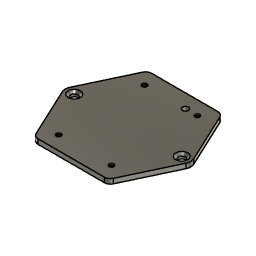
Metal Foot Pedal Bracket (Autodesk Fusion 360 design; units mm, degrees)
Autodesk Fusion 360 part; units mm, degrees
note: some values were not read from the file. Set by a fixed rule: which sketch regions a step uses.
sketch "Sketch1" plane through (0, 0, 0) normal (0, 0, 1) x (1, 0, 0)
  line L0 (22.1, 35.95) -> (-22.1, 35.95) construction
  line L1 (-22.1, 35.95) -> (-22.1, -35.95) construction
  line L2 (-22.1, -35.95) -> (22.1, -35.95) construction
  line L3 (22.1, -35.95) -> (22.1, 35.95) construction
  line L4 (22.1, 35.95) -> (-22.1, -35.95) construction
  line L5 (-22.1, 35.95) -> (22.1, -35.95) construction
  line L6 (23.8, 37.65) -> (-23.8, 37.65) construction
  line L7 (-23.8, 37.65) -> (-23.8, -37.65) construction
  line L8 (-23.8, -37.65) -> (23.8, -37.65) construction
  line L9 (23.8, -37.65) -> (23.8, 37.65) construction
  line L10 (23.8, 37.65) -> (-23.8, -37.65) construction
  line L11 (-23.8, 37.65) -> (23.8, -37.65) construction
  circle A0 centre (-22.1, 35.95) radius 1.7
  circle A1 centre (22.1, 35.95) radius 1.7
  circle A2 centre (-22.1, -35.95) radius 1.7
  circle A3 centre (22.1, -35.95) radius 1.7
  line L12 (-23.8, -34.25) -> (23.8, -34.25) construction
  line L13 (-20.4, -37.65) -> (-20.4, 37.65) construction
  line L14 (-23.8, 34.25) -> (23.8, 34.25) construction
  line L15 (20.4, 37.65) -> (20.4, -37.65) construction
  line L16 (31, 47.5) -> (-31, 47.5)
  line L17 (-31, 47.5) -> (-31, -47.5)
  line L18 (-31, -47.5) -> (31, -47.5)
  line L19 (31, -47.5) -> (31, 47.5)
  line L20 (31, 47.5) -> (-31, -47.5) construction
  line L21 (-31, 47.5) -> (31, -47.5) construction
  circle A4 centre (-45, 0) radius 3
  circle A5 centre (45, 0) radius 3
  circle A6 centre (-45, 0) radius 7.5
  circle A7 centre (45, 0) radius 7.5
  line L22 (-31, 47.5) -> (-51.7899, 3.1854)
  line L23 (-31, -47.5) -> (-51.7899, -3.1854)
  line L24 (31, -47.5) -> (51.7899, -3.1854)
  line L25 (31, 47.5) -> (51.7899, 3.1854)
  line L26 (45, 0) -> (0, 0) construction
  line L27 (0, 0) -> (-45, 0) construction
  circle A8 centre (12.1, 35.95) radius 2.5
  dimension "d1" = 75.3
  dimension "d2" = 68.5
  dimension "d3" = 40.8
  dimension "d4" = 47.6
  dimension "d5" = 95
  dimension "d6" = 62
  dimension "d7" = 6
  dimension "d8" = 6
  dimension "d9" = 15
  dimension "d10" = 15
  dimension "d11" = 45
  dimension "d12" = 45
  dimension "d13" = 10
  dimension "d14" = 5
  constraint horizontal L0
  constraint perpendicular L0 L1
  constraint parallel L0 L2
  constraint parallel L1 L3
  constraint coincident L4 L26.end
  constraint coincident L5 L26.end
  constraint coincident L26.end L27.start
  constraint horizontal L6
  constraint perpendicular L6 L7
  constraint parallel L6 L8
  constraint parallel L7 L9
  constraint coincident L10 L26.end
  constraint coincident L11 L26.end
  constraint coincident L0.end L1.start
  constraint coincident L0.start L3.end
  constraint coincident L1.end L2.start
  constraint coincident L2.end L3.start
  constraint tangent L8 A2
  constraint tangent L7 A2
  constraint tangent L8 A3
  constraint coincident L7 L12.start
  constraint coincident L9 L12.end
  constraint perpendicular L9 L12
  constraint coincident L8 L13.start
  constraint coincident L6 L13.end
  constraint coincident L7 L14.start
  constraint coincident L9 L14.end
  constraint perpendicular L9 L14
  constraint coincident L6 L15.start
  constraint coincident L8 L15.end
  constraint tangent A3 L15
  constraint vertical L15
  constraint tangent A1 L15
  constraint tangent L6 A1
  constraint tangent A1 L14
  constraint tangent A0 L14
  constraint tangent A0 L13
  constraint tangent A3 L12
  constraint tangent A2 L13
  constraint horizontal L16
  constraint perpendicular L16 L17
  constraint parallel L16 L18
  constraint parallel L17 L19
  constraint coincident L20 L26.end
  constraint coincident L21 L26.end
  constraint concentric A4 A6
  constraint concentric A5 A7
  constraint coincident A5.centre A7.centre
  constraint horizontal L26
  constraint coincident A4.centre A6.centre
  constraint parallel L26 L27
  constraint tangent A6 L22
  constraint tangent A6 L23
  constraint tangent A7 L24
  constraint tangent A7 L25
  constraint coincident A7 L25.end
  constraint coincident A7 L24.end
  constraint coincident A6 L23.end
  constraint coincident A6 L22.end
  constraint coincident L0 A8.centre
  measures "d1" distance of L6 L8
  measures "d2" distance of L12 L14
  measures "d3" distance of L13 L15
  measures "d4" distance of L7 L9
  measures "d5" distance of L16.end L17.end
  measures "d6" distance of L16.start L16.end
  measures "d7" diameter of A4
  measures "d8" diameter of A5
  measures "d9" diameter of A6
  measures "d10" diameter of A7
  measures "d11" distance of L26.end A4.centre
  measures "d12" distance of A5.centre L26.end
  measures "d13" distance of L0.start A8.centre
  measures "d14" diameter of A8
extrude "Extrude1" add sketch "Sketch1" along normal blind 4
fillet "Fillet1" radius 5 4 edges at (31, 47.5, 2) (-31, 47.5, 2) (31, -47.5, 2) (-31, -47.5, 2)
sketch "Sketch2" plane through (0, 0, 0) normal (0, 0, -1) x (1, 0, 0)
  circle A0 centre (45, 0) radius 3
  circle A1 centre (-22.1, 35.95) radius 1.7
  circle A2 centre (22.1, 35.95) radius 1.7
  circle A3 centre (-22.1, -35.95) radius 1.7
  circle A4 centre (-45, 0) radius 3
  circle A5 centre (22.1, -35.95) radius 1.7
  circle A6 centre (12.1, -35.95) radius 2.5
  arc A7 (-27.8228, 47.5) -> (-32.3494, 44.6236) centre (-27.8228, 42.5) ccw
  line L0 (-32.3494, 44.6236) -> (-51.7899, 3.1854)
  arc A8 (-51.7899, 3.1854) -> (-51.7899, -3.1854) centre (-45, 0) ccw
  line L1 (-51.7899, -3.1854) -> (-32.3494, -44.6236)
  arc A9 (-32.3494, -44.6236) -> (-27.8228, -47.5) centre (-27.8228, -42.5) ccw
  line L2 (-27.8228, -47.5) -> (27.8228, -47.5)
  arc A10 (27.8228, -47.5) -> (32.3494, -44.6236) centre (27.8228, -42.5) ccw
  line L3 (32.3494, -44.6236) -> (51.7899, -3.1854)
  arc A11 (51.7899, -3.1854) -> (51.7899, 3.1854) centre (45, 0) ccw
  line L4 (51.7899, 3.1854) -> (32.3494, 44.6236)
  arc A12 (32.3494, 44.6236) -> (27.8228, 47.5) centre (27.8228, 42.5) ccw
  line L5 (27.8228, 47.5) -> (-27.8228, 47.5)
  circle A13 centre (22.1, -35.95) radius 4.25
  circle A14 centre (-22.1, -35.95) radius 4.25
  circle A15 centre (-22.1, 35.95) radius 4.25
  circle A16 centre (22.1, 35.95) radius 4.25
  dimension "d19" = 8.5
  dimension "d20" = 8.5
  dimension "d21" = 8.5
  dimension "d22" = 8.5
  constraint concentric A5 A13
  constraint concentric A3 A14
  constraint concentric A1 A15
  constraint concentric A2 A16
  measures "d19" diameter of A16
  measures "d20" diameter of A15
  measures "d21" diameter of A14
  measures "d22" diameter of A13
extrude "Extrude2" cut sketch "Sketch2" against normal blind 2.4 contours A13 | A14 | A15 | A16
sketch "Sketch3" plane through (0, 0, 4) normal (0, 0, 1) x (-1, 0, 0)
  arc A0 (32.3494, 44.6236) -> (27.8228, 47.5) centre (27.8228, 42.5) ccw
  line L0 (27.8228, 47.5) -> (-27.8228, 47.5)
  arc A1 (-27.8228, 47.5) -> (-32.3494, 44.6236) centre (-27.8228, 42.5) ccw
  line L1 (-32.3494, 44.6236) -> (-51.7899, 3.1854)
  arc A2 (-51.7899, 3.1854) -> (-51.7899, -3.1854) centre (-45, 0) ccw
  line L2 (-51.7899, -3.1854) -> (-32.3494, -44.6236)
  arc A3 (-32.3494, -44.6236) -> (-27.8228, -47.5) centre (-27.8228, -42.5) ccw
  line L3 (-27.8228, -47.5) -> (27.8228, -47.5)
  arc A4 (27.8228, -47.5) -> (32.3494, -44.6236) centre (27.8228, -42.5) ccw
  line L4 (32.3494, -44.6236) -> (51.7899, -3.1854)
  arc A5 (51.7899, -3.1854) -> (51.7899, 3.1854) centre (45, 0) ccw
  line L5 (51.7899, 3.1854) -> (32.3494, 44.6236)
  circle A6 centre (-45, 0) radius 3
  circle A7 centre (22.1, 35.95) radius 1.7
  circle A8 centre (-22.1, 35.95) radius 1.7
  circle A9 centre (22.1, -35.95) radius 1.7
  circle A10 centre (45, 0) radius 3
  circle A11 centre (-22.1, -35.95) radius 1.7
  circle A12 centre (-12.1, -35.95) radius 2.5
  circle A13 centre (22.1, -35.95) radius 2
  circle A14 centre (-22.1, -35.95) radius 2
  circle A15 centre (-22.1, 35.95) radius 2
  circle A16 centre (22.1, 35.95) radius 2
  dimension "d25" = 4
  dimension "d26" = 4
  dimension "d27" = 4
  dimension "d28" = 4
  constraint concentric A9 A13
  constraint concentric A11 A14
  constraint concentric A8 A15
  constraint concentric A7 A16
  measures "d25" diameter of A13
  measures "d26" diameter of A14
  measures "d27" diameter of A15
  measures "d28" diameter of A16
extrude "Extrude3" cut sketch "Sketch3" against normal up to surface (1.6 mm away) contours A13 | A14 | A15 | A16
sketch "Sketch4" plane through (0, 0, 2.4) normal (0, 0, -1) x (1, 0, 0)
  circle A0 centre (-22.1, -35.95) radius 2
  circle A1 centre (-22.1, -35.95) radius 4.25
  circle A2 centre (-22.1, 35.95) radius 2
  circle A3 centre (-22.1, 35.95) radius 4.25
  circle A4 centre (22.1, 35.95) radius 2
  circle A5 centre (22.1, 35.95) radius 4.25
  circle A6 centre (22.1, -35.95) radius 2
  circle A7 centre (22.1, -35.95) radius 4.25
  line L0 (-24.1, 39.7) -> (-24.1, 32.2)
  line L1 (-20.1, 39.7) -> (-20.1, 32.2)
  line L2 (20.1, 39.7) -> (20.1, 32.2)
  line L3 (24.1, 39.7) -> (24.1, 32.2)
  line L4 (24.1, -32.2) -> (24.1, -39.7)
  line L5 (20.1, -32.2) -> (20.1, -39.7)
  line L6 (-20.1, -32.2) -> (-20.1, -39.7)
  line L7 (-24.1, -32.2) -> (-24.1, -39.7)
  constraint coincident A3 L0.start
  constraint coincident A3 L0.end
  constraint vertical L0
  constraint coincident A3 L1.start
  constraint coincident A3 L1.end
  constraint parallel L0 L1
  constraint coincident A5 L2.start
  constraint coincident A5 L2.end
  constraint parallel L1 L2
  constraint coincident A5 L3.start
  constraint coincident A5 L3.end
  constraint parallel L2 L3
  constraint coincident A7 L4.start
  constraint coincident A7 L4.end
  constraint parallel L3 L4
  constraint coincident A7 L5.start
  constraint parallel L4 L5
  constraint coincident A1 L6.start
  constraint coincident A1 L6.end
  constraint vertical L6
  constraint coincident A1 L7.start
  constraint coincident A1 L7.end
  constraint parallel L6 L7
  constraint tangent A0 L7
  constraint tangent A0 L6
  constraint tangent A6 L4
  constraint tangent A6 L5
  constraint coincident A7 L5.end
  constraint tangent A4 L2
  constraint tangent A4 L3
  constraint tangent A2 L1
  constraint tangent A2 L0
extrude "Extrude4" cut sketch "Sketch4" against normal blind 0.2 contours A0 A1 L6 L7 | A0 A1 L6 L7 | A2 A3 L0 L1 | A2 A3 L0 L1 | A4 A5 L2 L3 | A4 A5 L2 L3 | A6 A7 L4 L5 | A6 A7 L4 L5
sketch "Sketch5" plane through (0, 0, 2.6) normal (0, 0, -1) x (1, 0, 0)
  line L0 (-24.1, 39.7) -> (-24.1, 35.95)
  arc A0 (-20.1, 35.95) -> (-24.1, 35.95) centre (-22.1, 35.95) ccw
  line L1 (-20.1, 35.95) -> (-20.1, 39.7)
  arc A1 (-20.1, 39.7) -> (-24.1, 39.7) centre (-22.1, 35.95) ccw
  arc A2 (20.1, 32.2) -> (24.1, 32.2) centre (22.1, 35.95) ccw
  line L2 (24.1, 32.2) -> (24.1, 35.95)
  arc A3 (20.1, 35.95) -> (24.1, 35.95) centre (22.1, 35.95) ccw
  line L3 (20.1, 35.95) -> (20.1, 32.2)
  line L4 (20.1, 39.7) -> (20.1, 35.95)
  arc A4 (24.1, 35.95) -> (20.1, 35.95) centre (22.1, 35.95) ccw
  line L5 (24.1, 35.95) -> (24.1, 39.7)
  arc A5 (24.1, 39.7) -> (20.1, 39.7) centre (22.1, 35.95) ccw
  arc A6 (-24.1, 32.2) -> (-20.1, 32.2) centre (-22.1, 35.95) ccw
  line L6 (-20.1, 32.2) -> (-20.1, 35.95)
  arc A7 (-24.1, 35.95) -> (-20.1, 35.95) centre (-22.1, 35.95) ccw
  line L7 (-24.1, 35.95) -> (-24.1, 32.2)
  line L8 (20.1, -35.95) -> (20.1, -39.7)
  arc A8 (20.1, -39.7) -> (24.1, -39.7) centre (22.1, -35.95) ccw
  line L9 (24.1, -39.7) -> (24.1, -35.95)
  arc A9 (20.1, -35.95) -> (24.1, -35.95) centre (22.1, -35.95) ccw
  arc A10 (24.1, -32.2) -> (20.1, -32.2) centre (22.1, -35.95) ccw
  line L10 (20.1, -32.2) -> (20.1, -35.95)
  arc A11 (24.1, -35.95) -> (20.1, -35.95) centre (22.1, -35.95) ccw
  line L11 (24.1, -35.95) -> (24.1, -32.2)
  line L12 (-24.1, -35.95) -> (-24.1, -39.7)
  arc A12 (-24.1, -39.7) -> (-20.1, -39.7) centre (-22.1, -35.95) ccw
  line L13 (-20.1, -39.7) -> (-20.1, -35.95)
  arc A13 (-24.1, -35.95) -> (-20.1, -35.95) centre (-22.1, -35.95) ccw
  arc A14 (-20.1, -32.2) -> (-24.1, -32.2) centre (-22.1, -35.95) ccw
  line L14 (-24.1, -32.2) -> (-24.1, -35.95)
  arc A15 (-20.1, -35.95) -> (-24.1, -35.95) centre (-22.1, -35.95) ccw
  line L15 (-20.1, -35.95) -> (-20.1, -32.2)
  line L16 (-24.1, 37.95) -> (-20.1, 37.95)
  line L17 (-24.1, 33.95) -> (-20.1, 33.95)
  line L18 (20.1, 37.95) -> (24.1, 37.95)
  line L19 (20.1, 33.95) -> (24.1, 33.95)
  line L20 (20.1, -33.95) -> (24.1, -33.95)
  line L21 (24.1, -37.95) -> (20.1, -37.95)
  line L22 (-24.1, -33.95) -> (-20.1, -33.95)
  line L23 (-24.1, -37.95) -> (-20.1, -37.95)
  constraint coincident L0 L16.start
  constraint coincident L1 L16.end
  constraint perpendicular L1 L16
  constraint coincident L7 L17.start
  constraint coincident L6 L17.end
  constraint perpendicular L6 L17
  constraint coincident L4 L18.start
  constraint coincident L5 L18.end
  constraint perpendicular L5 L18
  constraint coincident L3 L19.start
  constraint coincident L2 L19.end
  constraint perpendicular L2 L19
  constraint coincident L10 L20.start
  constraint coincident L11 L20.end
  constraint perpendicular L11 L20
  constraint coincident L9 L21.start
  constraint coincident L8 L21.end
  constraint perpendicular L8 L21
  constraint coincident L14 L22.start
  constraint coincident L15 L22.end
  constraint perpendicular L15 L22
  constraint coincident L12 L23.start
  constraint coincident L13 L23.end
  constraint perpendicular L13 L23
  constraint tangent A15 L22
  constraint tangent A13 L23
  constraint tangent A9 L21
  constraint tangent A11 L20
  constraint tangent A3 L19
  constraint tangent A4 L18
  constraint tangent A7 L17
  constraint tangent A0 L16
extrude "Extrude5" cut sketch "Sketch5" against normal blind 0.2 contours L0 A0 L16 | A7 L7 L17 | A0 L1 L16 | L6 A7 L17 | A3 L3 L19 | L2 A3 L19 | L4 A4 L18 | A4 L5 L18 | L8 A9 L21 | L10 A11 L20 | L9 A9 L21 | A11 L11 L20 | L12 A13 L23 | L14 A15 L22 | L13 A13 L23 | A15 L15 L22
chamfer "Chamfer1" distance 2 angle 45 2 edges at (-47.797, 1.0848, 4) (42.203, 1.0848, 4)
